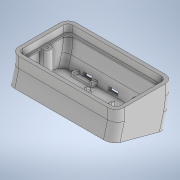
# Autodesk Inventor part: Case
Saved by Autodesk Inventor 2020 (Build 240168000, 168)
## iProperties
Created: 2021-01-03
Part Number: Case
Material: Generic
Document SubType Name: Modeling
Designer: user
Density: 1 g/cm^3
Appearance: Default
Author: user
Autodesk Inventor part; units mm, degrees
ref_plane "YZ Plane" through (0, 0, 0) normal (1, 0, 0) x (0, 1, 0)
ref_plane "XZ Plane" through (0, 0, 0) normal (0, 1, 0) x (-1, 0, 0)
ref_plane "XY Plane" through (0, 0, 0) normal (0, 0, 1) x (1, 0, 0)
sketch "Sketch1" plane through (0, 0, 0) normal (0, 0, 1) x (1, 0, 0)
  line L0 (0, 0) -> (82.1, 0)
  line L1 (82.1, 0) -> (82.1, 42.1)
  line L2 (82.1, 42.1) -> (0, 42.1)
  line L3 (0, 42.1) -> (0, 0)
  line L4 (-3, 45.1) -> (85.1, 45.1)
  line L5 (85.1, 45.1) -> (85.1, -3)
  line L6 (85.1, -3) -> (-3, -3)
  line L7 (-3, -3) -> (-3, 45.1)
  dimension "d0" = 82.1
  dimension "d1" = 42.1
  dimension "d2" = 3
  constraints: 16 end point, 4 parallel, 2 perpendicular, 1 horizontal, 3 other
  measures "d0" distance of L2.end L1.end
  measures "d1" distance of L1.end L0.end
  measures "d2" distance between parallel lines of L2 L4
extrude "Extrusion1" add sketch "Sketch1" along normal blind 6
sketch "Sketch2" plane through (0, 0, 0) normal (0, 0, -1) x (-1, 0, 0)
  line L0 (-85.1, -3) -> (-85.1, 45.1) projected
  line L1 (3, -3) -> (-85.1, -3) projected
  line L2 (-85.1, 45.1) -> (3, 45.1)
  line L3 (3, 45.1) -> (3, -3)
  line L4 (3, -3) -> (-85.1, -3)
  line L5 (-85.1, -3) -> (-85.1, 45.1)
  line L6 (-2, 40.1) -> (-80.1, 40.1)
  line L7 (-80.1, 40.1) -> (-80.1, 2)
  line L8 (-80.1, 2) -> (-2, 2)
  line L9 (-2, 2) -> (-2, 40.1)
  point P0 (0, 0)
  dimension "d5" = 5
  constraints: 16 end point, 4 parallel, 2 perpendicular, 1 horizontal, 3 other
  measures "d5" distance between parallel lines of L2 L6
extrude "Extrusion2" add sketch "Sketch2" along normal blind 3
sketch "Sketch3" plane through (0, 0, -3) normal (0, 0, -1) x (-1, 0, 0)
  line L0 (-85.1, 45.1) -> (3, 45.1) projected
  line L1 (3, 45.1) -> (3, -3) projected
  line L2 (-85.1, 45.1) -> (3, 45.1)
  line L3 (3, 45.1) -> (3, -3)
  line L4 (3, -3) -> (-85.1, -3)
  line L5 (-85.1, -3) -> (-85.1, 45.1)
  line L6 (-82.1, 42.1) -> (0, 42.1)
  line L7 (0, 42.1) -> (0, 0)
  line L8 (0, 0) -> (-82.1, 0)
  line L9 (-82.1, 0) -> (-82.1, 42.1)
  line L10 (-69.8862, -11) -> (-28.5374, -11)
  point P0 (0, 0)
  dimension "d8" = 3
  dimension "d9" = 8
  constraints: 18 end point, 4 parallel, 2 horizontal, 2 perpendicular, 3 other
  measures "d8" distance between parallel lines of L5 L9
  measures "d9" distance between parallel lines of L10 L4
revolve "Revolution1" add sketch "Sketch3" angle 15 about axis through (-3, -3, -3) along (-1, 0, 0)
sketch "Sketch4" plane through (85.1, 43.461, -15.4492) normal (0, -0.258819, -0.9659258) x (-1, 0, 0)
  line L0 (0, 0) -> (0, -48.1) projected
  line L1 (88.1, -48.1) -> (88.1, 0) projected
  line L2 (0, 0) -> (88.1, 0)
  line L3 (88.1, 0) -> (88.1, -48.1)
  line L4 (88.1, -48.1) -> (0, -48.1)
  line L5 (0, -48.1) -> (0, 0)
  line L6 (85.1, -3) -> (3, -3)
  line L7 (3, -3) -> (3, -45.1)
  line L8 (3, -45.1) -> (85.1, -45.1)
  line L9 (85.1, -45.1) -> (85.1, -3)
  point P0 (85.1, -45.9787)
  point P1 (0, -48.1)
  point P2 (88.1, 0)
  dimension "d11" = 3
  constraints: 16 end point, 4 parallel, 2 perpendicular, 1 horizontal, 3 other
  measures "d11" distance between parallel lines of L2 L6
extrude "Extrusion3" add sketch "Sketch4" along normal blind 10
sketch "Sketch5" plane through (85.1, 40.8728, -25.1085) normal (0, -0.258819, -0.9659258) x (-1, 0, 0)
  line L0 (88.1, 0) -> (0, 0) projected
  line L1 (0, -48.1) -> (88.1, -48.1) projected
  line L2 (0, 0) -> (88.1, 0)
  line L3 (88.1, 0) -> (88.1, -48.1)
  line L4 (88.1, -48.1) -> (0, -48.1)
  line L5 (0, -48.1) -> (0, 0)
  point P0 (85.1, -45.9787)
  point P1 (88.1, 0)
  point P2 (0, -48.1)
  constraints: 8 end point, 2 parallel, 1 horizontal, 1 perpendicular
extrude "Extrusion4" add sketch "Sketch5" along normal blind 3.2
fillet "Fillet1" radius 7 12 edges at (85.1, -4.7082, -9.3751) (85.1, -3, 1.5) (85.1, 41.7528, -21.8243) (85.1, 45.1, 1.5) (85.1, 44.6885, -9.2783) (-3, -4.7082, -9.3751) (-3, -3, 1.5) (-3, 44.6885, -9.2783) (-3, 40.4587, -26.6539) (-3, 42.1669, -20.2788) (-3, 45.1, -1.5) (-3, 45.1, 3)
fillet "Fillet2" radius 4 16 edges at (2, 40.1, -1.5) (0, 42.1, 3) (82.1, 42.1, 3) (80.1, 40.1, -1.5) (82.1, 39.2692, -19.5024) (82.1, 41.7142, -8.8867) (0, 39.2692, -19.5024) (0, 41.7142, -8.8867) (0, -0.0257, -3.3916) (0, -1.3963, -8.6061) (2, 2, -1.5) (0, 0, 3) (82.1, -0.0257, -3.3916) (82.1, -1.3963, -8.6061) (80.1, 2, -1.5) (82.1, 0, 3)
chamfer "Chamfer1" distance 2 angle 45 8 edges at (78.9284, 38.9284, -3) (80.1, 21.05, -3) (78.9284, 3.1716, -3) (41.05, 2, -3) (3.1716, 3.1716, -3) (2, 21.05, -3) (3.1716, 38.9284, -3) (41.05, 40.1, -3)
sketch "Sketch6" plane through (4, 43.461, -15.4492) normal (0, 0.9659258, -0.258819) x (1, 0, 0)
  line L0 (41.0625, 5.7) -> (33.0625, 5.7)
  line L1 (33.0625, 5.7) -> (33.0625, 8.7)
  line L2 (33.0625, 8.7) -> (41.0625, 8.7)
  line L3 (41.0625, 8.7) -> (41.0625, 5.7)
  line L4 (81.1, 0) -> (81.1, 13.2) projected
  line L5 (0, 13.2) -> (74.1, 13.2) projected
  point P0 (-4, -3.6742)
  dimension "d21" = 8
  dimension "d22" = 3
  dimension "d23" = 40.0375
  dimension "d24" = 4.5
  constraints: 8 end point, 2 parallel, 1 horizontal, 1 perpendicular
  measures "d21" distance of L1.end L2.end
  measures "d22" distance of L0.end L1.end
  measures "d23" distance between parallel lines of L3 L4
  measures "d24" distance between parallel lines of L5 L2
extrude "Extrusion5" cut sketch "Sketch6" against normal blind 6
sketch "Sketch7" plane through (85.1, 40.8728, -25.1085) normal (0, 0.258819, 0.9659258) x (1, 0, 0)
  line L0 (-7, -3) -> (-81.1, -3) projected
  line L1 (-53.15, -3) -> (-34.95, -3)
  line L2 (-34.95, -3) -> (-34.95, -36.075)
  line L3 (-34.95, -36.075) -> (-53.15, -36.075)
  line L4 (-53.15, -36.075) -> (-53.15, -3)
  line L5 (-88.1, -41.1) -> (-88.1, -7) projected
  line L6 (-55.15, -13) -> (-52.15, -13)
  line L7 (-52.15, -13) -> (-52.15, -16)
  line L8 (-52.15, -16) -> (-55.15, -16)
  line L9 (-55.15, -16) -> (-55.15, -13)
  line L10 (-35.95, -13) -> (-32.95, -13)
  line L11 (-32.95, -13) -> (-32.95, -16)
  line L12 (-32.95, -16) -> (-35.95, -16)
  line L13 (-35.95, -16) -> (-35.95, -13)
  line L14 (-45.55, -35.075) -> (-42.55, -35.075)
  line L15 (-42.55, -35.075) -> (-42.55, -38.075)
  line L16 (-42.55, -38.075) -> (-45.55, -38.075)
  line L17 (-45.55, -38.075) -> (-45.55, -35.075)
  point P0 (-85.1, -45.9787)
  dimension "d27" = 18.2
  dimension "d28" = 33.075
  dimension "d29" = 34.95
  dimension "d30" = 3
  dimension "d31" = 3
  dimension "d32" = 3
  dimension "d33" = 3
  dimension "d34" = 1
  dimension "d35" = 1
  dimension "d36" = 10
  dimension "d37" = 10
  dimension "d38" = 3
  dimension "d39" = 3
  dimension "d40" = 1
  dimension "d41" = 7.6
  constraints: 32 end point, 8 parallel, 4 horizontal, 4 perpendicular, 1 point on line
  measures "d27" distance of L2.end L3.end
  measures "d28" distance of L3.end L1.start
  measures "d29" distance between parallel lines of L5 L4
  measures "d30" distance of L7.end L8.end
  measures "d31" distance of L6.end L7.end
  measures "d32" distance of L11.end L12.end
  measures "d33" distance of L10.end L11.end
  measures "d34" distance between parallel lines of L7 L4
  measures "d35" distance between parallel lines of L2 L13
  measures "d36" distance between parallel lines of L0 L6
  measures "d37" distance between parallel lines of L0 L10
  measures "d38" distance of L15.end L16.end
  measures "d39" distance of L14.end L15.end
  measures "d40" distance between parallel lines of L3 L14
  measures "d41" distance between parallel lines of L17 L4
extrude "Extrusion6" add sketch "Sketch7" along normal blind 1 contours L10 L11 L12 L2 | L2 L12 L13 L10 | L6 L7 L8 L4 | L4 L8 L9 L6 | L15 L16 L17 L3 | L3 L17 L14 L15
sketch "Sketch8" plane through (85.1, 41.1317, -24.1425) normal (0, 0.258819, 0.9659258) x (1, 0, 0)
  line L0 (-55.15, -13) -> (-55.15, -16) projected
  line L1 (-55.15, -13) -> (-53.15, -13)
  line L2 (-53.15, -13) -> (-53.15, -16)
  line L3 (-53.15, -16) -> (-55.15, -16)
  line L4 (-55.15, -16) -> (-55.15, -13)
  line L5 (-32.95, -13) -> (-35.95, -13) projected
  line L6 (-32.95, -13) -> (-34.95, -13)
  line L7 (-34.95, -13) -> (-34.95, -16)
  line L8 (-34.95, -16) -> (-32.95, -16)
  line L9 (-32.95, -16) -> (-32.95, -13)
  line L10 (-45.55, -38.075) -> (-45.55, -35.075) projected
  line L11 (-45.55, -38.075) -> (-42.55, -38.075)
  line L12 (-42.55, -38.075) -> (-42.55, -36.075)
  line L13 (-42.55, -36.075) -> (-45.55, -36.075)
  line L14 (-45.55, -36.075) -> (-45.55, -38.075)
  point P0 (-85.1, -45.9787)
  dimension "d44" = 2
  dimension "d45" = 3
  dimension "d46" = 2
  dimension "d47" = 3
  dimension "d48" = 3
  dimension "d49" = 2
  constraints: 24 end point, 6 parallel, 3 horizontal, 3 perpendicular
  measures "d44" distance of L2.end L3.end
  measures "d45" distance of L1.end L2.end
  measures "d46" distance of L8.end L7.end
  measures "d47" distance of L7.end L6.end
  measures "d48" distance of L13.end L12.end
  measures "d49" distance of L12.end L11.end
extrude "Extrusion7" add sketch "Sketch8" along normal blind 2
chamfer "Chamfer2" distance 1 angle 45 3 edges at (31.95, 27.6434, -18.4578) (50.15, 27.6434, -18.4578) (41.05, 6.8035, -12.8738)
sketch "Sketch9" plane through (0, 0, 0) normal (0, 0, 1) x (1, 0, 0)
  circle A0 centre (3.575, 21.05) radius 1
  circle A1 centre (3.575, 21.05) radius 3
  line L0 (76.1, 40.1) -> (6, 40.1) projected
  line L1 (2, 36.1) -> (2, 6) projected
  line L2 (3.575, 24.05) -> (2, 24.05)
  line L3 (3.575, 18.05) -> (2, 18.05)
  line L4 (2, 24.05) -> (0, 24.05)
  line L5 (0, 34.1114) -> (0, 1.1733) projected
  line L6 (2, 18.05) -> (0, 18.05)
  line L7 (0, 24.05) -> (0, 18.05)
  line L8 (41.05, 37.8955) -> (41.05, 27.7746)
  circle A2 centre (78.525, 21.05) radius 1
  circle A3 centre (78.525, 21.05) radius 3
  line L9 (78.525, 24.05) -> (80.1, 24.05)
  line L10 (78.525, 18.05) -> (80.1, 18.05)
  line L11 (80.1, 24.05) -> (82.1, 24.05)
  line L12 (80.1, 18.05) -> (82.1, 18.05)
  line L13 (82.1, 24.05) -> (82.1, 18.05)
  line L14 (82.1, 1.1733) -> (82.1, 34.1114) projected
  point P0 (0, 0)
  point P1 (0, 18.05)
  dimension "d55" = 2
  dimension "d56" = 2
  dimension "d57" = 19.05
  dimension "d58" = 1.575
  dimension "d61" = 41.05
  constraints: 22 end point, 7 symmetric about line, 4 centre point, 4 point on circle, 3 perpendicular, 3 point on line, 2 horizontal, 2 tangent, 1 collinear, 1 vertical, 2 other
  measures "d55" diameter of A0
  measures "d56" radial gap between concentric circles of A0 A1
  measures "d57" distance from line of A0.centre L0
  measures "d58" distance from line of L1 A0.centre
  measures "d61" distance between parallel lines of L8 L5
extrude "Extrusion8" add sketch "Sketch9" against normal blind 20
sketch "Sketch10" plane through (4, 43.461, -15.4492) normal (0, 0.9659258, -0.258819) x (1, 0, 0)
  line L0 (19.0625, 8.7) -> (12.0625, 8.7)
  line L1 (12.0625, 8.7) -> (12.0625, 5.7)
  line L2 (12.0625, 5.7) -> (19.0625, 5.7)
  line L3 (19.0625, 5.7) -> (19.0625, 8.7)
  line L4 (33.0625, 8.7) -> (41.0625, 8.7) projected
  line L5 (33.0625, 5.7) -> (33.0625, 8.7) projected
  point P0 (-4, -3.6742)
  dimension "d62" = 7
  dimension "d63" = 3
  dimension "d64" = 0
  dimension "d65" = 14
  constraints: 8 end point, 2 parallel, 1 horizontal, 1 perpendicular
  measures "d62" distance of L2.end L1.end
  measures "d63" distance of L1.end L0.end
  measures "d64" distance between parallel lines of L4 L0
  measures "d65" distance between parallel lines of L5 L3
extrude "Extrusion9" cut sketch "Sketch10" against normal blind 10
sketch "Sketch11" plane through (85.1, 40.8728, -25.1085) normal (0, 0.258819, 0.9659258) x (1, 0, 0)
  line L0 (-7, -3) -> (-81.1, -3) projected
  line L1 (-71.9125, -3) -> (-59.1625, -3)
  line L2 (-59.1625, -3) -> (-59.1625, -7.4999)
  line L3 (-59.1625, -7.4999) -> (-71.9125, -7.4999)
  line L4 (-71.9125, -7.4999) -> (-71.9125, -3)
  line L5 (-73.9125, -3) -> (-57.1625, -3)
  line L6 (-57.1625, -3) -> (-57.1625, -8)
  line L7 (-57.1625, -8) -> (-73.9125, -8)
  line L8 (-73.9125, -8) -> (-73.9125, -3)
  point P0 (-85.1, -45.9787)
  point P1 (-69.0375, -3)
  point P2 (-57.1625, -3)
  dimension "d68" = 12.75
  dimension "d69" = 2.875
  dimension "d70" = 2
  dimension "d71" = 2
  dimension "d72" = 5
  constraints: 16 end point, 4 parallel, 2 horizontal, 2 perpendicular, 2 point on line
  measures "d68" distance of L2.end L3.end
  measures "d69" distance from line of L4 point (-69.038, -3)
  measures "d70" distance between parallel lines of L4 L8
  measures "d71" distance between parallel lines of L6 L2
  measures "d72" distance between parallel lines of L7 L0
extrude "Extrusion10" add sketch "Sketch11" along normal blind 1.5
sketch "Sketch12" plane through (85.1, 41.2611, -23.6596) normal (0, 0.258819, 0.9659258) x (1, 0, 0)
  line L0 (-73.9125, -3) -> (-57.1625, -3) projected
  line L1 (-71.9125, -3) -> (-59.1625, -3)
  line L2 (-59.1625, -3) -> (-59.1625, -8)
  line L3 (-59.1625, -8) -> (-71.9125, -8)
  line L4 (-71.9125, -8) -> (-71.9125, -3)
  line L5 (-73.9125, -3) -> (-73.9125, -8) projected
  line L6 (-57.1625, -8) -> (-57.1625, -3) projected
  line L7 (-73.9125, -8) -> (-57.1625, -8) projected
  line L8 (-73.9125, -8) -> (-73.9125, -3) projected
  line L9 (-73.9125, -3) -> (-71.9125, -3)
  line L10 (-71.9125, -3) -> (-71.9125, -8)
  line L11 (-71.9125, -8) -> (-73.9125, -8)
  line L12 (-73.9125, -8) -> (-73.9125, -3)
  line L13 (-59.1625, -3) -> (-57.1625, -3)
  line L14 (-57.1625, -3) -> (-57.1625, -8)
  line L15 (-57.1625, -8) -> (-59.1625, -8)
  line L16 (-59.1625, -8) -> (-59.1625, -3)
  point P0 (-85.1, -45.9787)
  point P1 (-59.1625, -3)
  point P2 (-71.9125, -8)
  dimension "d75" = 2
  dimension "d76" = 2
  dimension "d77" = 0
  constraints: 24 end point, 6 parallel, 3 horizontal, 3 perpendicular, 1 point on line
  measures "d75" distance between parallel lines of L5 L4
  measures "d76" distance between parallel lines of L6 L2
  measures "d77" distance between parallel lines of L7 L3
extrude "Extrusion11" add sketch "Sketch12" along normal blind 2 contours L0 L4 L7 L5 | L0 L6 L7 L2
sketch "Sketch13" plane through (85.1, 40.0446, -28.1994) normal (0, -0.258819, -0.9659258) x (-1, 0, 0)
  circle A0 centre (80.1, -40.1) radius 6.5
  circle A1 centre (80.1, -8) radius 6.5
  circle A2 centre (8, -40.1) radius 6.5
  circle A3 centre (8, -8) radius 6.5
  line L0 (7, -48.1) -> (81.1, -48.1) projected
  line L1 (88.1, -41.1) -> (88.1, -7) projected
  line L2 (81.1, 0) -> (7, 0) projected
  line L3 (0, -7) -> (0, -41.1) projected
  point P0 (85.1, -45.9787)
  dimension "d80" = 13
  dimension "d81" = 13
  dimension "d82" = 13
  dimension "d83" = 13
  dimension "d84" = 8
  dimension "d85" = 8
  dimension "d86" = 8
  dimension "d87" = 8
  dimension "d88" = 8
  dimension "d89" = 8
  dimension "d90" = 8
  dimension "d91" = 8
  constraints: 4 centre point
  measures "d80" diameter of A0
  measures "d81" diameter of A1
  measures "d82" diameter of A2
  measures "d83" diameter of A3
  measures "d84" distance from line of L0 A0.centre
  measures "d85" distance from line of L1 A0.centre
  measures "d86" distance from line of L2 A1.centre
  measures "d87" distance from line of A1.centre L1
  measures "d88" distance from line of L0 A2.centre
  measures "d89" distance from line of L3 A2.centre
  measures "d90" distance from line of L3 A3.centre
  measures "d91" distance from line of L2 A3.centre
extrude "Extrusion12" cut sketch "Sketch13" against normal blind 2.6
body "Solid1"
